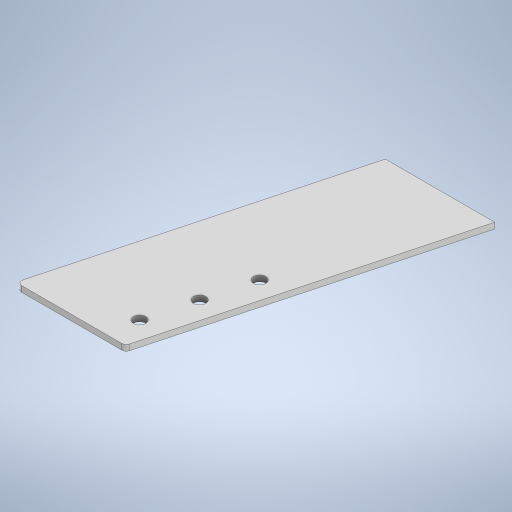
# Autodesk Inventor part: держатель полки 1
Saved by Autodesk Inventor 2024.2 (Build 282272000, 272)
## iProperties
Created: 2024-06-15
Part Number: держатель полки 1
Material: Generic
Document SubType Name: Sheet Metal
Designer: admin
Density: 1 g/cm^3
Sheet Metal Rule: Default
Appearance: Default
Author: admin
Autodesk Inventor part; units mm, degrees
ref_plane "YZ Plane" through (0, 0, 0) normal (1, 0, 0) x (0, 1, 0)
ref_plane "XZ Plane" through (0, 0, 0) normal (0, 1, 0) x (-1, 0, 0)
ref_plane "XY Plane" through (0, 0, 0) normal (0, 0, 1) x (1, 0, 0)
sketch "Sketch1" plane through (0, 0, 0) normal (0, 0, 1) x (1, 0, 0)
  line L0 (-150, 0) -> (150, 0)
  line L1 (150, 0) -> (150, -200) construction
  line L2 (150, -200) -> (-150, -200)
  line L3 (-150, -200) -> (-150, 0) construction
  line L4 (-150, 0) -> (-203.5898, -200)
  line L5 (-203.5898, -200) -> (-150, -200)
  line L6 (150, 0) -> (203.5898, -200)
  line L7 (203.5898, -200) -> (150, -200)
  line L8 (0, 0) -> (-53.5898, -200)
  line L9 (-150, 0) -> (-96.4102, 200)
  line L10 (-96.4102, 200) -> (53.5898, 200)
  line L11 (53.5898, 200) -> (0, 0)
  dimension "d0" = 300
  dimension "d1" = 200
  dimension "d2" = 15
  dimension "d25" = 200
  measures "d0" distance of L1.end L2.end
  measures "d1" distance of L0.end L1.end
  measures "d2" angle of L3 L4
  measures "d25" distance between parallel lines of L0 L10
extrude "Plate1" add sketch "Sketch1" along normal blind 8 contours L9 L10 L11 L0 | L0 L8 L2 L5 L4
sketch "Sketch3" plane through (0, 0, 8) normal (0, 0, 1) x (1, 0, 0)
  line L0 (-53.5898, -200) -> (-203.5898, -200) projected
  line L1 (-203.5898, -200) -> (-96.4102, 200) projected
  line L2 (-39.0968, -30) -> (-73.9302, -160) construction
  line L3 (-203.5898, -200) -> (-150, 0) projected
  line L4 (53.5898, 200) -> (-53.5898, -200) projected
  line L5 (-96.4102, 200) -> (53.5898, 200) projected
  point P0 (0, 0)
  point P1 (-56.5135, -95)
  point P2 (0, 0)
  dimension "d13" = 40
  dimension "d26" = 30
  dimension "d27" = 30
  constraints: 2 coincident, 2 end point, 2 midpoint, 1 parallel
  measures "d13" distance from line of L0 point (-73.93, -160)
  measures "d26" distance between parallel lines of L4 L2
  measures "d27" vertical distance of point (-39.097, -30) point (0, 0)
hole "Hole1" at (-39.0968, -30, 8) at (-56.5135, -95, 8) at (-73.9302, -160, 8) direction (0, 0, -1) diameter 17 end through all
fillet "Corner Round1" radius 6 2 edges at (-203.5898, -200, 4) (-53.5898, -200, 4)
equation "\"d9\" = Thickness"
equation "\"d3\" = Thickness"
equation "\"BendRadius\" = Thickness"
equation "\"BendReliefWidth\" = Thickness"
equation "\"BendReliefDepth\" = 0.5 * Thickness"
equation "\"CornerReliefSize\" = 4 * Thickness"
equation "\"MinimumRemnant\" = 2 * Thickness"
equation "\"TransitionRadius\" = BendRadius"
equation "\"JacobiRadiusSize\" = BendRadius"
equation "\"GapSize\" = Thickness"
equation "\"Thickness\" = 8"
body "Solid1"
